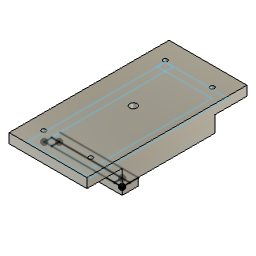
Tripod_Connector (Autodesk Fusion 360 design; units mm, degrees)
Autodesk Fusion 360 part; units mm, degrees
note: some values were not read from the file. Set by a fixed rule: which face or edge a step refers to.
sketch "Sketch1" plane through (0, 0, 0) normal (0, 0, 1) x (1, 0, 0)
  line L0 (-25, 35) -> (19, 35)
  line L1 (19, 35) -> (19, -79)
  line L2 (19, -79) -> (-25, -79)
  line L3 (-25, -79) -> (-25, 35)
  line L4 (-25, 35) -> (-32.5, 35)
  line L5 (-32.5, 35) -> (-32.5, 42.5)
  line L6 (-32.5, 42.5) -> (-25, 42.5)
  line L7 (-25, 42.5) -> (-25, 35)
  line L8 (-32.5, 42.5) -> (26.5, 42.5)
  line L9 (26.5, 42.5) -> (26.5, -86.5)
  line L10 (26.5, -86.5) -> (-32.5, -86.5)
  line L11 (-32.5, -86.5) -> (-32.5, 42.5)
  dimension "d1" = 44
  dimension "d2" = 114
  dimension "d3" = 7.5
  dimension "d4" = 7.5
  dimension "d5" = 59
  dimension "d6" = 129
  constraint horizontal L0
  constraint vertical L1
  constraint horizontal L2
  constraint vertical L3
  constraint horizontal L4
  constraint vertical L5
  constraint horizontal L6
  constraint vertical L7
  constraint horizontal L8
  constraint vertical L9
  constraint horizontal L10
  constraint vertical L11
  measures "d1" distance of L0.start L0.end
  measures "d2" distance of L0.start L2.end
  measures "d3" distance of L0.start L4.end
  measures "d4" distance of L0.start L6.end
  measures "d5" distance of L5.end L8.end
  measures "d6" distance of L5.end L10.end
extrude "Extrude1" add sketch "Sketch1" along normal blind 7 contours L0 L1 L2 L3 | L4 L7 L8 L9 L10 L11 | L4 L5 L6 L7 L8 L11 makes body 1
sketch "Sketch2" plane through (0, 0, 0) normal (0, 0, 1) x (1, 0, 0)
  circle A0 centre (-25, -79) radius 7
  circle A1 centre (19, -79) radius 7
  circle A2 centre (19, 35) radius 7
  circle A3 centre (-25, 35) radius 7
  point P0 (-25, -79)
  point P1 (19, -79)
  point P2 (19, 35)
  point P3 (-25, 35)
  dimension "d9" = 14
  dimension "d10" = 14
  dimension "d11" = 14
  dimension "d12" = 14
  constraint coincident P0 A0.centre
  constraint coincident P1 A1.centre
  constraint coincident P2 A2.centre
  constraint coincident P3 A3.centre
  measures "d9" diameter of A0
  measures "d10" diameter of A1
  measures "d11" diameter of A2
  measures "d12" diameter of A3
extrude "Extrude2" cut sketch "Sketch2" along normal blind 4 contours A0 bodies 1
extrude "Extrude3" cut sketch "Sketch2" along normal blind 4 contours A1 bodies 1
extrude "Extrude4" cut sketch "Sketch2" along normal blind 4 contours A3 bodies 1
extrude "Extrude5" cut sketch "Sketch2" along normal blind 4 contours A2 bodies 1
sketch "Sketch3" plane through (0, 0, 0) normal (0, 0, 1) x (1, 0, 0)
hole "Hole1" at (-25, -79, 4) direction (0, 0, 1) diameter 4 depth 10 tip angle 118 bodies 1
hole "Hole2" at (19, -79, 4) direction (0, 0, 1) diameter 4 depth 10 tip angle 118 bodies 1
hole "Hole3" at (19, 35, 4) direction (0, 0, 1) diameter 4 depth 10 tip angle 118 bodies 1
hole "Hole4" at (-25, 35, 4) direction (0, 0, 1) diameter 4 depth 10 tip angle 118 bodies 1
extrude "Extrude6" add 1 faces at (-12.8333, 42.5, 2.3333) along direction (0, 1, 0) blind 10.5 on bodies 1 bodies 1
extrude "Extrude7" add 1 faces at (6.8333, -86.5, 2.3333) along direction (0, -1, 0) blind 10.5 on bodies 1 bodies 1
sketch "Sketch4" plane through (0, 0, 0) normal (0, 0, -1) x (1, 0, 0)
  circle A0 centre (19, -35) radius 7
  circle A1 centre (-25, -35) radius 7
  circle A2 centre (19, 79) radius 7
  circle A3 centre (-25, 79) radius 7
  line L0 (-32.5, 97) -> (-32.5, -53)
  line L1 (-32.5, -53) -> (26.5, -53)
  line L2 (26.5, -53) -> (26.5, 97)
  line L3 (26.5, 97) -> (-32.5, 97)
  line L4 (-32.5, -53) -> (26.5, -53)
  line L5 (26.5, -53) -> (26.5, 17)
  line L6 (26.5, 17) -> (-32.5, 17)
  line L7 (-32.5, 17) -> (-32.5, -53)
  line L8 (-32.5, 17) -> (-3, 17)
  line L9 (26.5, 17) -> (-3, 17)
  dimension "d37" = 70
  constraint horizontal L4
  constraint vertical L5
  constraint horizontal L6
  constraint vertical L7
  constraint coincident L0.end L1.start
  constraint midpoint L6 L8.end
  measures "d37" distance of L0.end L6.end
hole "Hole5" at (-3, -17, 0) direction (0, 0, 1) diameter 7 depth 10 tip angle 118 bodies 1
sketch "Sketch5" plane through (0, 0, 0) normal (0, 0, -1) x (1, 0, 0)
  line L0 (26.5, 17) -> (-32.5, 17)
  line L1 (-32.5, 17) -> (-32.5, -23)
  line L2 (-32.5, -23) -> (26.5, -23)
  line L3 (26.5, -23) -> (26.5, 17)
  point P0 (26.5, 17)
  dimension "d41" = 59
  dimension "d42" = 40
  constraint horizontal L0
  constraint vertical L1
  constraint horizontal L2
  constraint vertical L3
  constraint coincident P0 L0.start
  measures "d41" distance of P0 L0.end
  measures "d42" distance of P0 L2.end
sketch "Sketch6" plane through (0, 0, 7) normal (0, 0, 1) x (-1, 0, 0)
  circle A0 centre (3, 17) radius 3.5
  circle A1 centre (25, -35) radius 2
  circle A2 centre (-19, -35) radius 2
  circle A3 centre (-19, 79) radius 2
  circle A4 centre (25, 79) radius 2
  line L0 (-26.5, 97) -> (-26.5, -53)
  line L1 (-26.5, -53) -> (32.5, -53)
  line L2 (32.5, -53) -> (32.5, 97)
  line L3 (32.5, 97) -> (-26.5, 97)
  line L4 (-26.5, 17) -> (32.5, 17)
  line L5 (32.5, 17) -> (32.5, 57)
  line L6 (32.5, 57) -> (-26.5, 57)
  line L7 (-26.5, 57) -> (-26.5, 17)
  line L8 (32.5, 57) -> (-26.5, 57)
  line L9 (-26.5, 57) -> (-26.5, 64)
  line L10 (-26.5, 64) -> (32.5, 64)
  line L11 (32.5, 64) -> (32.5, 57)
  point P0 (-26.5, 17)
  dimension "d43" = 40
  dimension "d44" = 7
  constraint horizontal L4
  constraint vertical L5
  constraint horizontal L6
  constraint vertical L7
  constraint coincident L2 L5.end
  constraint coincident P0 L4.start
  constraint horizontal L8
  constraint vertical L9
  constraint horizontal L10
  constraint vertical L11
  constraint coincident L0 L9.end
  measures "d43" distance of P0 L6.end
  measures "d44" distance of L5.end L10.end
sketch "Sketch7" plane through (-32.5, 0, 0) normal (-1, 0, 0) x (0, -1, 0)
  line L0 (-53, 0) -> (97, 0)
  line L1 (97, 0) -> (97, 7)
  line L2 (97, 7) -> (-53, 7)
  line L3 (-53, 7) -> (-53, 0)
  line L4 (57, 7) -> (64, 7)
  line L5 (64, 7) -> (64, 0)
  line L6 (64, 0) -> (57, 0)
  line L7 (57, 0) -> (57, 7)
  point P0 (57, 7)
  constraint horizontal L4
  constraint vertical L5
  constraint horizontal L6
  constraint vertical L7
  constraint coincident L0 L5.end
  constraint coincident P0 L4.start
sketch "Sketch8" plane through (26.5, 0, 0) normal (1, 0, 0) x (0, 1, 0)
  line L0 (-97, 0) -> (53, 0)
  line L1 (53, 0) -> (53, 7)
  line L2 (53, 7) -> (-97, 7)
  line L3 (-97, 7) -> (-97, 0)
  line L4 (-64, 7) -> (-57, 7)
  line L5 (-57, 7) -> (-57, 0)
  line L6 (-57, 0) -> (-64, 0)
  line L7 (-64, 0) -> (-64, 7)
  point P0 (-64, 7)
  point P1 (-57, 0)
  constraint horizontal L4
  constraint vertical L5
  constraint horizontal L6
  constraint vertical L7
  constraint coincident P1 L5.end
  constraint coincident P0 L4.start
extrude "Extrude8" add sketch "Sketch8" along normal blind 7 separate body contours L0 L2 L4 L5 L6 L7 | L0 L1 L2 L5 makes body 2
sketch "Sketch9" plane through (0, 0, 0) normal (0, 0, -1) x (1, 0, 0)
  line L0 (-32.5, 57) -> (26.5, 57)
  line L1 (26.5, 57) -> (26.5, 64)
  line L2 (26.5, 64) -> (-32.5, 64)
  line L3 (-32.5, 64) -> (-32.5, 57)
  point P0 (-32.5, 57)
  point P1 (26.5, 64)
  constraint horizontal L0
  constraint vertical L1
  constraint horizontal L2
  constraint vertical L3
  constraint coincident P1 L1.end
  constraint coincident P0 L0.start
extrude "Extrude9" add sketch "Sketch7" along normal blind 7 separate body contours L0 L2 L3 L7 | L0 L2 L4 L5 L6 L7 makes body 3
sketch "Sketch10" plane through (0, 0, 0) normal (0, 0, -1) x (1, 0, 0)
  line L0 (26.5, 64) -> (26.5, -53)
  line L1 (26.5, -53) -> (33.5, -53)
  line L2 (33.5, -53) -> (33.5, 64)
  line L3 (33.5, 64) -> (26.5, 64)
  line L4 (-32.5, -53) -> (-39.5, -53)
  line L5 (-39.5, -53) -> (-39.5, -23)
  line L6 (-39.5, -23) -> (-32.5, -23)
  line L7 (-32.5, -23) -> (-32.5, -53)
  line L8 (33.5, -53) -> (26.5, -53)
  line L9 (26.5, -53) -> (26.5, -23)
  line L10 (26.5, -23) -> (33.5, -23)
  line L11 (33.5, -23) -> (33.5, -53)
  line L12 (-32.5, -23) -> (-39.5, -23)
  line L13 (-39.5, -23) -> (-39.5, 64)
  line L14 (-39.5, 64) -> (-32.5, 64)
  line L15 (-32.5, 64) -> (-32.5, -23)
  line L16 (33.5, -23) -> (26.5, -23)
  line L17 (26.5, -23) -> (26.5, 64)
  line L18 (26.5, 64) -> (33.5, 64)
  line L19 (33.5, 64) -> (33.5, -23)
  point P0 (-32.5, -53)
  point P1 (26.5, -23)
  point P2 (-39.5, 64)
  dimension "d49" = 30
  constraint horizontal L4
  constraint vertical L5
  constraint horizontal L6
  constraint vertical L7
  constraint coincident P0 L4.start
  constraint horizontal L8
  constraint vertical L9
  constraint horizontal L10
  constraint vertical L11
  constraint coincident P1 L9.end
  constraint coincident L1.end L2.start
  constraint horizontal L12
  constraint vertical L13
  constraint horizontal L14
  constraint vertical L15
  constraint coincident P2 L13.end
  constraint horizontal L16
  constraint vertical L17
  constraint horizontal L18
  constraint vertical L19
  constraint coincident L0.start L3.end
  measures "d49" distance of P0 L6.end
extrude "Extrude10" add sketch "Sketch9" sketch "Sketch10" along normal blind 15 of sketch 2 contours L0 L2 L3 L10 L16 L17 L18 L19 | L6 L12 L13 L14 L15 bodies 1 2 3
extrude "Extrude11" add sketch "Sketch8" along normal blind 7 contours L0 L2 L3 L7 bodies 1
extrude "Extrude12" add sketch "Sketch7" along normal blind 7 contours L0 L1 L2 L5 bodies 1
extrude "Extrude13" add 1 faces at (-3, -58.4478, 7) along direction (0, 0, 1) blind 2 on bodies 1 bodies 1
sketch "Sketch11" plane through (0, 0, -15) normal (0, 0, -1) x (1, 0, 0)
  line L0 (-32.5, 57) -> (26.5, 57)
  line L1 (26.5, 57) -> (26.5, -23)
  line L2 (26.5, -23) -> (33.5, -23)
  line L3 (33.5, -23) -> (33.5, 64)
  line L4 (33.5, 64) -> (-39.5, 64)
  line L5 (-39.5, 64) -> (-39.5, -23)
  line L6 (-39.5, -23) -> (-32.5, -23)
  line L7 (-32.5, -23) -> (-32.5, 57)
  line L8 (-32.5, 57) -> (-39.5, 57)
  line L9 (-39.5, 57) -> (-39.5, 64)
  line L10 (-39.5, 64) -> (-32.5, 64)
  line L11 (-32.5, 64) -> (-32.5, 57)
  line L12 (26.5, 57) -> (33.5, 57)
  line L13 (33.5, 57) -> (33.5, 64)
  line L14 (33.5, 64) -> (26.5, 64)
  line L15 (26.5, 64) -> (26.5, 57)
  line L16 (26.5, 57) -> (-32.5, 57)
  line L17 (-32.5, 57) -> (-32.5, 64)
  line L18 (-32.5, 64) -> (26.5, 64)
  line L19 (26.5, 64) -> (26.5, 57)
  line L20 (33.5, 57) -> (-39.5, 57)
  line L21 (-39.5, 57) -> (-39.5, 49)
  line L22 (-39.5, 49) -> (33.5, 49)
  line L23 (33.5, 49) -> (33.5, 57)
  dimension "d58" = 8
  constraint horizontal L8
  constraint vertical L9
  constraint horizontal L10
  constraint vertical L11
  constraint coincident L4.end L5.start
  constraint coincident L0.start L7.end
  constraint horizontal L12
  constraint vertical L13
  constraint horizontal L14
  constraint vertical L15
  constraint coincident L3.end L4.start
  constraint coincident L0.end L1.start
  constraint horizontal L16
  constraint vertical L17
  constraint horizontal L18
  constraint vertical L19
  constraint horizontal L20
  constraint vertical L21
  constraint horizontal L22
  constraint vertical L23
  measures "d58" distance of L12.end L22.end
extrude "Extrude14" add sketch "Sketch11" along normal blind 7 separate body contours L0 L4 L11 L15 L16 L17 L18 L19 L20 | L4 L5 L8 L9 L10 L11 L17 L20 | L3 L4 L12 L13 L14 L15 L19 L20 makes body 4
extrude "Extrude15" add 3 faces at (-34.8333, -57, -17.3333) (-12.8333, -57, -17.3333) (28.8333, -57, -17.3333) along direction (0, 1, 0) blind 8 on bodies 4 bodies 1 4
